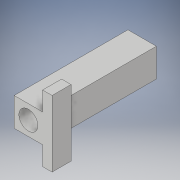
# Autodesk Inventor part: new cup 1
Saved by Autodesk Inventor 2017.3 (Build 213256000, 256)
## iProperties
Created: 2018-08-30
Part Number: new cup 1
Material: Generic
Document SubType Name: Modeling
Designer: Mac
Density: 1 g/cm^3
Appearance: Default
Author: Mac
Autodesk Inventor part; units mm, degrees
ref_plane "YZ Plane" through (0, 0, 0) normal (1, 0, 0) x (0, 1, 0)
ref_plane "XZ Plane" through (0, 0, 0) normal (0, 1, 0) x (-1, 0, 0)
ref_plane "XY Plane" through (0, 0, 0) normal (0, 0, 1) x (1, 0, 0)
sketch "Sketch1" plane through (0, 0, 0) normal (0, 0, 1) x (1, 0, 0)
  line L0 (0, 0) -> (-9.525, 0)
  line L1 (-9.525, 0) -> (-9.525, 9.525)
  line L2 (-9.525, 9.525) -> (0, 9.525)
  line L3 (0, 9.525) -> (0, 0)
  dimension "d0" = 9.525
  dimension "d1" = 9.525
  constraints: 8 end point, 2 parallel, 1 horizontal, 1 perpendicular
  measures "d0" distance of L1.end L2.end
  measures "d1" distance of L0.end L1.end
extrude "Extrusion1" add sketch "Sketch1" along normal blind 38.1
sketch "Sketch2" plane through (0, 0, 38.1) normal (0, 0, 1) x (1, 0, 0)
  circle A0 centre (-4.7625, 4.7625) radius 3.175
  point P0 (0, 0)
  dimension "d4" = 6.35
  constraints: 1 centre point
  measures "d4" diameter of A0
extrude "Extrusion2" cut sketch "Sketch2" against normal blind 38.1
sketch "Sketch3" plane through (0, 0, 0) normal (1, 0, 0) x (0, 0, -1)
  line L0 (-38.1, -6.35) -> (-31.75, -6.35)
  line L1 (-31.75, -6.35) -> (-31.75, 15.875)
  line L2 (-31.75, 15.875) -> (-38.1, 15.875)
  line L3 (-38.1, 15.875) -> (-38.1, -6.35)
  point P0 (0, 0)
  dimension "d7" = 6.35
  dimension "d8" = 22.225
  constraints: 8 end point, 2 parallel, 1 horizontal, 1 perpendicular
  measures "d7" distance of L2.end L1.end
  measures "d8" distance of L1.end L0.end
extrude "Extrusion3" add sketch "Sketch3" along normal blind 3.175
body "Solid1"
